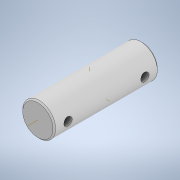
# Autodesk Inventor part: crankshaft pin
Saved by Autodesk Inventor 2021.1 (Build 251245000, 245)
## iProperties
Created: 2020-08-31
Part Number: crankshaft pin
Material: Generic
Document SubType Name: Sheet Metal
Designer: Vamshi
Density: 1 g/cm^3
Sheet Metal Rule: Default
Appearance: Default
Author: Vamshi
Autodesk Inventor part; units mm, degrees
ref_plane "YZ Plane" through (0, 0, 0) normal (1, 0, 0) x (0, 1, 0)
ref_plane "XZ Plane" through (0, 0, 0) normal (0, 1, 0) x (-1, 0, 0)
ref_plane "XY Plane" through (0, 0, 0) normal (0, 0, 1) x (1, 0, 0)
sketch "Sketch1" plane through (0, 0, 0) normal (0, 0, 1) x (1, 0, 0)
  circle A0 centre (0, 0) radius 15.24
  dimension "d0" = 30.48
  constraints: 1 centre point, 1 coincident
  measures "d0" diameter of A0
extrude "Extrusion1" add sketch "Sketch1" along normal mid plane 96.52
sketch "Sketch2" plane through (0, 0, 0) normal (1, 0, 0) x (0, 1, 0)
  line L0 (15.24, -48.26) -> (-15.24, -48.26) projected
  line L1 (-15.24, -48.26) -> (-15.24, 48.26) projected
  line L2 (-15.24, 48.26) -> (15.24, 48.26) projected
  line L3 (15.24, 48.26) -> (15.24, -48.26) projected
  line L4 (-15.24, -48.26) -> (15.24, -48.26) projected
  line L5 (15.24, 48.26) -> (-15.24, 48.26) projected
  line L6 (-21.336, 0) -> (21.336, 0) projected
  line L7 (0, -67.564) -> (0, 67.564) projected
  circle A0 centre (0, 35.56) radius 3.81
  circle A1 centre (0, -35.56) radius 3.81
  point P0 (0, 0)
  dimension "d3" = 7.62
  dimension "d4" = 7.62
  dimension "d5" = 12.7
  dimension "d6" = 12.7
  constraints: 2 centre point, 2 point on line
  measures "d3" diameter of A0
  measures "d4" diameter of A1
  measures "d5" distance from line of L2 A0.centre
  measures "d6" distance from line of L0 A1.centre
extrude "Extrusion2" cut sketch "Sketch2" against normal through all both and the other way through all contours A1 L7 | L7 A1 | A0 L7 | L7 A0
chamfer "Chamfer1" distance 1.27 angle 45 2 edges at (-15.24, 0, 48.26) (-15.24, 0, -48.26) measured on face at (-15.24, 0, -47.76) measured on face at (-15.24, 0, 47.76)
equation "\"BendRadius\" = Thickness"
equation "\"BendReliefWidth\" = Thickness"
equation "\"BendReliefDepth\" = 0.5 * Thickness"
equation "\"CornerReliefSize\" = 4 * Thickness"
equation "\"MinimumRemnant\" = 2 * Thickness"
equation "\"TransitionRadius\" = BendRadius"
equation "\"JacobiRadiusSize\" = BendRadius"
equation "\"GapSize\" = Thickness"
equation "\"Thickness\" = 3.048"
body "Solid1"
